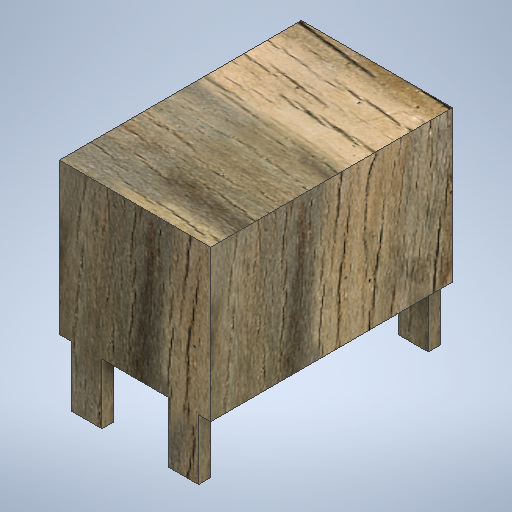
# Autodesk Inventor part: Caja
Saved by Autodesk Inventor 2025.2 (Build 292293000, 293)
## iProperties
Created: 2025-11-06
Part Number: Caja
Material: Genérico
Document SubType Name: Modeling
Designer: Dax
Density: 1 g/cm^3
Appearance: Madera de deriva
Author: Dax
Autodesk Inventor part; units mm, degrees
ref_plane "YZ Plane" through (0, 0, 0) normal (1, 0, 0) x (0, 1, 0)
ref_plane "XZ Plane" through (0, 0, 0) normal (0, 1, 0) x (-1, 0, 0)
ref_plane "XY Plane" through (0, 0, 0) normal (0, 0, 1) x (1, 0, 0)
sketch "Boceto1" plane through (0, 0, 0) normal (0, 1, 0) x (-1, 0, 0)
  line L0 (-25, 40) -> (25, 40)
  line L1 (25, 40) -> (25, -40)
  line L2 (25, -40) -> (-25, -40)
  line L3 (-25, -40) -> (-25, 40)
  line L4 (-25, 40) -> (25, -40) construction
  line L5 (25, 40) -> (-25, -40) construction
  point P0 (0, 0)
  dimension "d0" = 50
  dimension "d1" = 80
  constraints: 12 end point, 2 midpoint, 2 parallel, 1 horizontal, 1 perpendicular
  measures "d0" distance of L1.end L2.end
  measures "d1" distance of L0.end L1.end
extrude "Extrusión1" add sketch "Boceto1" along normal blind 50
sketch "Boceto2" plane through (0, 0, 0) normal (0, -1, 0) x (1, 0, 0)
  line L0 (-25, 40) -> (25, 40) projected
  line L1 (21, 40) -> (11, 40)
  line L2 (11, 40) -> (11, 36)
  line L3 (11, 36) -> (21, 36)
  line L4 (21, 36) -> (21, 40)
  line L5 (-25, -40) -> (25, -40)
  line L6 (21, -40) -> (11, -40)
  line L7 (11, -40) -> (11, -36)
  line L8 (11, -36) -> (21, -36)
  line L9 (21, -36) -> (21, -40)
  line L10 (25, 40) -> (-25, 40)
  line L11 (-11, 40) -> (-11, 36)
  line L12 (-11, 36) -> (-21, 36)
  line L13 (-21, 36) -> (-21, 40)
  line L14 (-21, -36) -> (-21, -40)
  line L15 (-11, -40) -> (-11, -36)
  line L16 (-11, -36) -> (-21, -36)
  line L17 (25, -40) -> (-25, -40)
  point P0 (0, 0)
  dimension "d6" = 4
  constraints: 34 end point, 8 point on line, 3 perpendicular
  measures "d6" distance of L1.end L2.end
extrude "Extrusión2" add sketch "Boceto2" along normal blind 20
